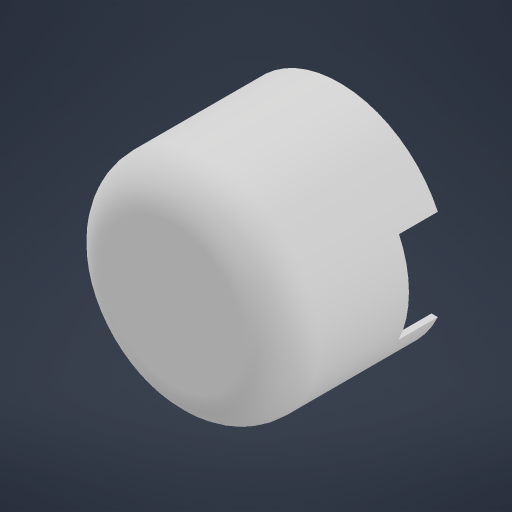
# Autodesk Inventor part: Elbow Cap
Saved by Autodesk Inventor 2024.1 (Build 281209000, 209)
## iProperties
Created: 2023-09-12
Part Number: Elbow Cap
Material: Generic
Document SubType Name: Modeling
Designer: User
Density: 1 g/cm^3
Appearance: Default
Author: User
Autodesk Inventor part; units mm, degrees
ref_plane "YZ Plane" through (0, 0, 0) normal (1, 0, 0) x (0, 1, 0)
ref_plane "XZ Plane" through (0, 0, 0) normal (0, 1, 0) x (-1, 0, 0)
ref_plane "XY Plane" through (0, 0, 0) normal (0, 0, 1) x (1, 0, 0)
sketch "Sketch1" plane through (0, 0, 0) normal (0, 0, 1) x (1, 0, 0)
  point P0 (0, 0)
sketch "Sketch2" plane through (0, 0, 0) normal (0, 0, 1) x (1, 0, 0)
  line L0 (-13, 0) -> (-10.5, 0) construction
  line L1 (-12.7574, 0) -> (-12.7574, 3.75)
  line L2 (-12.7574, 0) -> (-9.0074, 0) construction
  line L3 (-12.7574, 3.75) -> (-12.7574, -3.75)
  line L4 (13.5, 0) -> (13.5, 6)
  line L5 (13.5, 0) -> (19.5, 0) construction
  line L6 (13.5, 6) -> (13.5, -6)
  line L7 (13.7477, -6) -> (12.0934, -6)
  line L8 (13.7477, 6) -> (12.0934, 6)
  line L9 (-12.9687, 3.75) -> (-14.5237, 3.75)
  line L10 (-12.9687, -3.75) -> (-14.5237, -3.75)
  arc A0 (12.0934, 6) -> (-12.9687, 3.75) centre (0, 0) ccw
  arc A1 (-12.9687, -3.75) -> (12.0934, -6) centre (0, 0) ccw
  arc A2 (-13.7477, -3.75) -> (12.9253, -6) centre (0, 0) ccw
  arc A3 (12.9253, 6) -> (-13.7477, 3.75) centre (0, 0) ccw
  dimension "d41" = 3.75
  dimension "d42" = 90
  dimension "d43" = 7.5
  dimension "d45" = 6
  dimension "d46" = 90
  constraints: 22 end point, 8 point on circle, 7 point on line, 5 horizontal, 4 centre point, 2 perpendicular, 2 vertical, 1 coincident, 1 midpoint, 1 parallel
  measures "d41" distance of L1.start L1.end
  measures "d42" angle of L2 L1
  measures "d43" distance of L1.end L3.end
  measures "d45" distance of L4.start L4.end
  measures "d46" angle of L5 L4
extrude "Extrusion1" add sketch "Sketch2" along normal blind 5
sketch "Sketch4" plane through (0, 0, 5) normal (0, 0, 1) x (1, 0, 0)
  circle A0 centre (0, 0) radius 13.5
  circle A1 centre (0, 0) radius 14.25
  dimension "d23" = 27
  dimension "d24" = 28.5
  constraints: 2 centre point, 2 coincident
  measures "d23" diameter of A0
  measures "d24" diameter of A1
extrude "Extrusion3" add sketch "Sketch4" along normal blind 12
sketch "Sketch5" plane through (0, 0, 17) normal (0, 0, 1) x (1, 0, 0)
  circle A0 centre (0, 0) radius 14.25
  dimension "d12" = 28.5
  constraints: 1 centre point, 1 coincident
  measures "d12" diameter of A0
extrude "Extrusion4" add sketch "Sketch5" along normal blind 5
fillet "Fillet2" radius 5 1 edges at (-14.25, 0, 22)
fillet "Fillet3" radius 0.2 6 edges at (-14.25, 0, 5) (13.9149, -3.0723, 5) (13.9149, 3.0723, 5) (13.1436, -3.0813, 5) (13.1436, 3.0813, 5) (-13.5, 0, 5)
body "Solid1"
